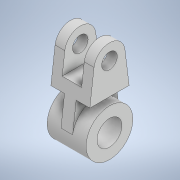
# Autodesk Inventor part: Exercise04
Saved by Autodesk Inventor 2021 (Build 250183000, 183)
## iProperties
Created: 2022-03-22
Part Number: Exercise04
Material: Generic
Document SubType Name: Modeling
Designer: User
Density: 1 g/cm^3
Appearance: Default
Author: User
Autodesk Inventor part; units mm, degrees
ref_plane "YZ Plane" through (0, 0, 0) normal (1, 0, 0) x (0, 1, 0)
ref_plane "XZ Plane" through (0, 0, 0) normal (0, 1, 0) x (-1, 0, 0)
sketch "Sketch1" plane through (0, 0, 0) normal (1, 0, 0) x (0, 1, 0)
  circle A0 centre (0, 0) radius 30
  circle A1 centre (0, 0) radius 16
  dimension "d0" = 60
  dimension "d1" = 32
  constraints: 2 centre point, 2 coincident
  measures "d0" diameter of A0
  measures "d1" diameter of A1
extrude "Extrusion1" add sketch "Sketch1" along normal blind 50
sketch "Sketch2" plane through (50, 0, 0) normal (1, 0, 0) x (0, 0, -1)
  circle A0 centre (0, 80) radius 10
  circle A1 centre (0, 80) radius 20
  line L0 (-19.8431, 82.5) -> (-29.7647, 3.75)
  line L1 (19.8431, 82.5) -> (29.7647, 3.75)
  circle A2 centre (0, 0) radius 30 projected
  line L2 (-25.1976, 40) -> (25.1976, 40)
  dimension "d4" = 20
  dimension "d5" = 40
  dimension "d6" = 80
  dimension "d7" = 40
  constraints: 6 end point, 4 point on circle, 4 tangent, 2 centre point, 2 point on line, 1 coincident, 1 horizontal, 1 vertical alignment
  measures "d4" diameter of A0
  measures "d5" diameter of A1
  measures "d6" distance of point (0, 0) A0.centre
  measures "d7" distance from line of L2 A0.centre
extrude "Extrusion2" add sketch "Sketch2" against normal blind 50 contours A1 | A1 L1 L2 L0
sketch "Sketch3" plane through (0, 0, 0) normal (0, 0, 1) x (1, 0, 0)
  line L0 (12.5, 115.7738) -> (37.5, 115.7738)
  line L1 (37.5, 115.7738) -> (37.5, 55.7738)
  line L2 (37.5, 55.7738) -> (12.5, 55.7738)
  line L3 (12.5, 55.7738) -> (12.5, 115.7738)
  line L4 (0, 100) -> (0, 82.5) projected
  line L5 (0, 70) -> (0, 90) projected
  line L6 (50, 90) -> (50, 70) projected
  line L7 (0, 80.7738) -> (50, 80.7738)
  point P0 (0, 0)
  dimension "d10" = 12.5
  dimension "d11" = 25
  dimension "d12" = 25
  dimension "d13" = 60
  constraints: 10 end point, 2 horizontal, 2 parallel, 2 perpendicular, 2 point on line
  measures "d10" distance between parallel lines of L4 L3
  measures "d11" distance of L0.start L0.end
  measures "d12" distance between parallel lines of L7 L2
  measures "d13" distance of L0.end L1.end
extrude "Extrusion3" cut sketch "Sketch3" along normal through all both and the other way through all
ref_plane "Work Plane1" through (25, 0, 0) normal (1, 0, 0) x (0, 0, -1)
sketch "Sketch4" plane through (25, 0, 0) normal (1, 0, 0) x (0, 0, -1)
  line L0 (25.1976, 40) -> (29.7647, 3.75)
  line L1 (-25.1976, 40) -> (-29.7647, 3.75)
  circle A0 centre (0, 0) radius 30 projected
  line L2 (25.1976, 40) -> (-25.1976, 40) projected
  constraints: 4 end point, 2 coincident, 2 point on circle, 2 tangent
extrude "Extrusion4" add sketch "Sketch4" along normal mid plane 15 contours L0 A0 L1 L2
body "Solid1"
